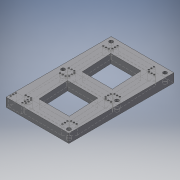
# Autodesk Inventor part: Segment
Saved by Autodesk Inventor 2016 SP2 (Build 200236200, 236)
## iProperties
Created: 2018-06-10
Part Number: Segment
Material: Generisch
Document SubType Name: Modeling
Designer: Nils
Density: 1 g/cm^3
Appearance: Vorgabe
Author: Nils
Autodesk Inventor part; units mm, degrees
ref_plane "YZ Plane" through (0, 0, 0) normal (1, 0, 0) x (0, 1, 0)
ref_plane "XZ Plane" through (0, 0, 0) normal (0, 1, 0) x (-1, 0, 0)
ref_plane "XY Plane" through (0, 0, 0) normal (0, 0, 1) x (1, 0, 0)
sketch "Skizze1" plane through (0, 0, 0) normal (0, 0, 1) x (1, 0, 0)
  line L0 (42.6168, 71.3457) -> (42.6168, -71.3457) projected
  line L1 (42.6168, -71.3457) -> (-42.6168, -71.3457) projected
  line L2 (-42.6168, -71.3457) -> (-42.6168, 71.3457) projected
  line L3 (-42.6168, 71.3457) -> (42.6168, 71.3457) projected
  line L4 (-27.6168, 66.3457) -> (22.3832, 66.3457) construction
  line L5 (22.3832, 56.3457) -> (-27.6168, 56.3457) construction
  line L6 (-28.3239, 55.6386) -> (-25.7071, 5.7071) construction
  line L7 (25.7071, 5.7071) -> (23.0903, 55.6386) construction
  line L8 (-25, 5) -> (25, 5) construction
  line L9 (25, -5) -> (-25, -5) construction
  line L10 (-25.7071, -5.7071) -> (-23.0903, -55.6386) construction
  line L11 (-22.3832, -56.3457) -> (27.6168, -56.3457) construction
  line L12 (27.6168, -66.3457) -> (-22.3832, -66.3457) construction
  line L13 (28.3239, -55.6386) -> (25.7071, -5.7071) construction
  line L14 (-22.5832, -56.1457) -> (27.8168, -56.1457)
  line L15 (27.8168, -56.1457) -> (27.8168, -66.5457)
  line L16 (27.8168, -66.5457) -> (-22.5832, -66.5457)
  line L17 (-22.5832, -66.5457) -> (-22.5832, -56.1457)
  line L18 (-25.2, 5.2) -> (25.2, 5.2)
  line L19 (25.2, 5.2) -> (25.2, -5.2)
  line L20 (25.2, -5.2) -> (-25.2, -5.2)
  line L21 (-25.2, -5.2) -> (-25.2, 5.2)
  line L22 (-27.8168, 66.5457) -> (22.5832, 66.5457)
  line L23 (22.5832, 66.5457) -> (22.5832, 56.1457)
  line L24 (22.5832, 56.1457) -> (-27.8168, 56.1457)
  line L25 (-27.8168, 56.1457) -> (-27.8168, 66.5457)
  line L26 (-25.4969, 5.5178) -> (-28.1346, 55.8488)
  line L27 (-28.1346, 55.8488) -> (-38.5204, 55.3045)
  line L28 (-38.5204, 55.3045) -> (-35.8827, 4.9736)
  line L29 (-35.8827, 4.9736) -> (-25.4969, 5.5178)
  line L30 (-25.5178, -5.4969) -> (-35.9036, -6.0412)
  line L31 (-35.9036, -6.0412) -> (-33.2659, -56.3721)
  line L32 (-33.2659, -56.3721) -> (-22.8801, -55.8278)
  line L33 (-22.8801, -55.8278) -> (-25.5178, -5.4969)
  line L34 (28.1346, -55.8488) -> (38.5204, -55.3045)
  line L35 (38.5204, -55.3045) -> (35.8827, -4.9736)
  line L36 (35.8827, -4.9736) -> (25.4969, -5.5178)
  line L37 (25.4969, -5.5178) -> (28.1346, -55.8488)
  line L38 (22.8801, 55.8278) -> (25.5178, 5.4969)
  line L39 (25.5178, 5.4969) -> (35.9178, 6.042)
  line L40 (35.9178, 6.042) -> (33.2801, 56.3729)
  line L41 (33.2801, 56.3729) -> (22.8801, 55.8278)
  circle A0 centre (-34.6168, -63.3457) radius 4 construction
  line L42 (-24.4168, -57.8457) -> (-41.4168, -57.8457)
  line L43 (-41.4168, -57.8457) -> (-41.4168, -68.8457)
  line L44 (-41.4168, -68.8457) -> (-24.4168, -68.8457)
  line L45 (-24.4168, -68.8457) -> (-24.4168, -57.8457)
  line L46 (20.7354, -10.2) -> (-20.2645, -10.2)
  line L47 (-20.2645, -10.2) -> (-18.1186, -51.1457)
  line L48 (-18.1186, -51.1457) -> (22.8813, -51.1457)
  line L49 (22.8813, -51.1457) -> (20.7354, -10.2)
  line L50 (-22.8813, 51.1457) -> (-20.7354, 10.2)
  line L51 (-22.8813, 51.1457) -> (18.1186, 51.1457)
  line L52 (20.2645, 10.2) -> (-20.7354, 10.2)
  line L53 (18.1186, 51.1457) -> (20.2645, 10.2)
  point P0 (0, 0)
  dimension "d0" = 0.2
  dimension "d1" = 0.2
  dimension "d2" = 0.2
  dimension "d3" = 0.2
  dimension "d4" = 0.2
  dimension "d5" = 0.2
  dimension "d6" = 0.2
  dimension "d7" = 0.2
  dimension "d8" = 0.2
  dimension "d9" = 0.2
  dimension "d10" = 0.2
  dimension "d11" = 0.2
  dimension "d12" = 0.2
  dimension "d13" = 0.2
  dimension "d14" = 0.2
  dimension "d17" = 10.4
  dimension "d18" = 10.4
  dimension "d19" = 10.4
  dimension "d21" = 50.4
  dimension "d22" = 50.4
  dimension "d23" = 50.4
  dimension "d24" = 0.2
  dimension "d25" = 0.2
  dimension "d26" = 0.2
  dimension "d28" = 90
  dimension "d29" = 50.4
  dimension "d30" = 0.2
  dimension "d31" = 0.2
  dimension "d32" = 10.4
  dimension "d35" = 17
  dimension "d36" = 11
  dimension "d37" = 5.5
  dimension "d38" = 1.2
  dimension "d49" = 5
  dimension "d50" = 5
  dimension "d51" = 5
  dimension "d52" = 5
  dimension "d54" = 5
  dimension "d56" = 5
  dimension "d57" = 5
  dimension "d58" = 5
  constraints: 80 end point, 21 parallel, 10 perpendicular, 7 horizontal
  measures "d0" distance between parallel lines of L14 L11
  measures "d1" distance between parallel lines of L12 L16
  measures "d2" distance from line of L17 L12.end
  measures "d3" distance from line of L12.start L15
  measures "d4" distance between parallel lines of L9 L20
  measures "d5" distance between parallel lines of L8 L18
  measures "d6" distance from line of L19 L8.end
  measures "d7" distance from line of L9.end L21
  measures "d8" distance between parallel lines of L5 L24
  measures "d9" distance between parallel lines of L22 L4
  measures "d10" distance from line of L23 L5.start
  measures "d11" distance from line of L25 L5.end
  measures "d12" distance between parallel lines of L13 L37
  measures "d13" distance between parallel lines of L33 L10
  measures "d14" distance between parallel lines of L26 L6
  measures "d17" distance between parallel lines of L35 L37
  measures "d18" distance between parallel lines of L31 L33
  measures "d19" distance between parallel lines of L28 L26
  measures "d21" distance of L34.end L35.end
  measures "d22" distance of L30.end L31.end
  measures "d23" distance of L27.end L28.end
  measures "d24" distance from line of L32 L10.end
  measures "d25" distance from line of L34 L13.start
  measures "d26" distance from line of L29 L6.end
  measures "d28" angle of L40 L39
  measures "d29" distance of L39.end L40.end
  measures "d30" distance from line of L39 L7.start
  measures "d31" distance between parallel lines of L7 L38
  measures "d32" horizontal distance of L38.end L39.end
  measures "d35" distance of L43.end L44.end
  measures "d36" distance between parallel lines of L44 L42
  measures "d37" distance from line of L44 A0.centre
  measures "d38" distance between parallel lines of L2 L43
  measures "d49" distance between parallel lines of L49 L37
  measures "d50" distance between parallel lines of L33 L47
  measures "d51" distance between parallel lines of L14 L48
  measures "d52" distance between parallel lines of L20 L46
  measures "d54" distance between parallel lines of L26 L50
  measures "d56" distance between parallel lines of L53 L38
  measures "d57" distance between parallel lines of L24 L51
  measures "d58" distance between parallel lines of L52 L18
extrude "Extrusion1" add sketch "Skizze1" along normal blind 11 contours L0 L1 L2 L3 | L45 L44 L43 L42
sketch "Skizze2" plane through (0, 0, 0) normal (0, 0, -1) x (-1, 0, 0)
  line L0 (22.3832, -56.3457) -> (27.3832, -61.3457) construction
  line L1 (27.3832, -61.3457) -> (22.3832, -66.3457) construction
  line L2 (22.3832, -66.3457) -> (-27.6168, -66.3457) construction
  line L3 (-27.6168, -66.3457) -> (-32.6168, -61.3457) construction
  line L4 (-32.6168, -61.3457) -> (-27.6168, -56.3457) construction
  line L5 (-27.6168, -56.3457) -> (22.3832, -56.3457) construction
  line L6 (-25, 5) -> (25, 5) construction
  line L7 (25, 5) -> (30, 0) construction
  line L8 (30, 0) -> (25, -5) construction
  line L9 (25, -5) -> (-25, -5) construction
  line L10 (-25, -5) -> (-30, 0) construction
  line L11 (-30, 0) -> (-25, 5) construction
  line L12 (-22.3832, 66.3457) -> (27.6168, 66.3457) construction
  line L13 (27.6168, 66.3457) -> (32.6168, 61.3457) construction
  line L14 (32.6168, 61.3457) -> (27.6168, 56.3457) construction
  line L15 (27.6168, 56.3457) -> (-22.3832, 56.3457) construction
  line L16 (-22.3832, 56.3457) -> (-27.3832, 61.3457) construction
  line L17 (-27.3832, 61.3457) -> (-22.3832, 66.3457) construction
  line L18 (23.0903, -55.6386) -> (25.7071, -5.7071) construction
  line L19 (25.7071, -5.7071) -> (30.7071, -0.7071) construction
  line L20 (30.7071, -0.7071) -> (35.7071, -5.7071) construction
  line L21 (35.7071, -5.7071) -> (33.0903, -55.6386) construction
  line L22 (33.0903, -55.6386) -> (28.0903, -60.6386) construction
  line L23 (28.0903, -60.6386) -> (23.0903, -55.6386) construction
  line L24 (-30.7071, -0.7071) -> (-25.7071, -5.7071) construction
  line L25 (-25.7071, -5.7071) -> (-28.3239, -55.6386) construction
  line L26 (-28.3239, -55.6386) -> (-33.3239, -60.6386) construction
  line L27 (-33.3239, -60.6386) -> (-38.3239, -55.6386) construction
  line L28 (-38.3239, -55.6386) -> (-35.7071, -5.7071) construction
  line L29 (-35.7071, -5.7071) -> (-30.7071, -0.7071) construction
  line L30 (35.7071, 5.7071) -> (30.7071, 0.7071) construction
  line L31 (30.7071, 0.7071) -> (25.7071, 5.7071) construction
  line L32 (25.7071, 5.7071) -> (28.3239, 55.6386) construction
  line L33 (28.3239, 55.6386) -> (33.3239, 60.6386) construction
  line L34 (33.3239, 60.6386) -> (38.3239, 55.6386) construction
  line L35 (38.3239, 55.6386) -> (35.7071, 5.7071) construction
  line L36 (-23.0903, 55.6386) -> (-25.7071, 5.7071) construction
  line L37 (-25.7071, 5.7071) -> (-30.7071, 0.7071) construction
  line L38 (-30.7071, 0.7071) -> (-35.7071, 5.7071) construction
  line L39 (-35.7071, 5.7071) -> (-33.0903, 55.6386) construction
  line L40 (-33.0903, 55.6386) -> (-28.0903, 60.6386) construction
  line L41 (-28.0903, 60.6386) -> (-23.0903, 55.6386) construction
  circle A0 centre (34.6168, -63.3457) radius 4 construction
  line L42 (-42.6168, -71.3457) -> (42.6168, -71.3457) construction
  line L43 (42.6168, -71.3457) -> (42.6168, 71.3457) construction
  line L44 (42.6168, 71.3457) -> (-42.6168, 71.3457) construction
  line L45 (-42.6168, 71.3457) -> (-42.6168, -71.3457) construction
  line L46 (-25.4969, -5.5178) -> (-30.7071, -0.3077)
  line L47 (-30.7071, -0.3077) -> (-35.3984, -4.9989)
  line L48 (-25.4969, -5.5178) -> (-35.8827, -4.9736) projected
  line L49 (-35.3984, -4.9989) -> (-35.8827, -4.9736)
  line L50 (-38.5204, -55.3045) -> (-28.1346, -55.8488) projected
  line L51 (-28.1346, -55.8488) -> (-33.3239, -61.038)
  line L52 (-33.3239, -61.038) -> (-38.5471, -55.8148)
  line L53 (-38.5471, -55.8148) -> (-38.5204, -55.3045)
  line L54 (-33.2801, 56.3729) -> (-22.8801, 55.8278) construction
  line L55 (-22.8801, 55.8278) -> (-25.5178, 5.4969) construction
  line L56 (-25.5178, 5.4969) -> (-35.9178, 6.042) construction
  line L57 (-35.9178, 6.042) -> (-33.2801, 56.3729) construction
  line L58 (-25.4969, -5.5178) -> (-28.1346, -55.8488) construction
  line L59 (-28.1346, -55.8488) -> (-38.5204, -55.3045) construction
  line L60 (-38.5204, -55.3045) -> (-35.8827, -4.9736) construction
  line L61 (-35.8827, -4.9736) -> (-25.4969, -5.5178) construction
  line L62 (22.8801, -55.8278) -> (25.5178, -5.4969) construction
  line L63 (25.5178, -5.4969) -> (35.9036, -6.0412) construction
  line L64 (35.9036, -6.0412) -> (33.2659, -56.3721) construction
  line L65 (33.2659, -56.3721) -> (22.8801, -55.8278) construction
  line L66 (35.8827, 4.9736) -> (25.4969, 5.5178) construction
  line L67 (25.4969, 5.5178) -> (28.1346, 55.8488) construction
  line L68 (28.1346, 55.8488) -> (38.5204, 55.3045) construction
  line L69 (38.5204, 55.3045) -> (35.8827, 4.9736) construction
  line L70 (-22.5832, 56.1457) -> (-22.5832, 66.5457) construction
  line L71 (-22.5832, 66.5457) -> (27.8168, 66.5457) construction
  line L72 (27.8168, 66.5457) -> (27.8168, 56.1457) construction
  line L73 (27.8168, 56.1457) -> (-22.5832, 56.1457) construction
  line L74 (-25.2, -5.2) -> (-25.2, 5.2) construction
  line L75 (-25.2, 5.2) -> (25.2, 5.2) construction
  line L76 (25.2, 5.2) -> (25.2, -5.2) construction
  line L77 (25.2, -5.2) -> (-25.2, -5.2) construction
  line L78 (-27.8168, -66.5457) -> (-27.8168, -56.1457) construction
  line L79 (-27.8168, -56.1457) -> (22.5832, -56.1457) construction
  line L80 (22.5832, -56.1457) -> (22.5832, -66.5457) construction
  line L81 (22.5832, -66.5457) -> (-27.8168, -66.5457) construction
  line L82 (-42.6168, 71.3457) -> (-42.6168, -71.3457) construction
  line L83 (-42.6168, -71.3457) -> (42.6168, -71.3457) construction
  line L84 (42.6168, -71.3457) -> (42.6168, 71.3457) construction
  line L85 (42.6168, 71.3457) -> (-42.6168, 71.3457) construction
  line L86 (22.5832, -56.1457) -> (-27.8168, -56.1457) projected
  line L87 (-27.8168, -56.1457) -> (-33.0168, -61.3457)
  line L88 (-33.0168, -61.3457) -> (-27.8168, -66.5457)
  line L89 (-27.8168, -66.5457) -> (22.5832, -66.5457) projected
  line L90 (-27.8168, -66.5457) -> (-27.8168, -56.1457)
  line L91 (22.5832, -66.5457) -> (22.5832, -56.1457) projected
  line L92 (22.5832, -66.5457) -> (27.7832, -61.3457)
  line L93 (27.7832, -61.3457) -> (22.5832, -56.1457)
  line L94 (22.5832, -56.1457) -> (22.5832, -66.5457)
  line L95 (22.8801, -55.8278) -> (33.2659, -56.3721) projected
  line L96 (22.8801, -55.8278) -> (28.0906, -61.0383)
  line L97 (28.0906, -61.0383) -> (32.7821, -56.3468)
  line L98 (33.2659, -56.3721) -> (35.9036, -6.0412) projected
  line L99 (33.2659, -56.3721) -> (32.7821, -56.3468)
  line L100 (35.9036, -6.0412) -> (25.5178, -5.4969) projected
  line L101 (25.5178, -5.4969) -> (30.7071, -0.3077)
  line L102 (30.7071, -0.3077) -> (35.9303, -5.5309)
  line L103 (35.9303, -5.5309) -> (35.9036, -6.0412)
  line L104 (35.9036, -6.0412) -> (25.5178, -5.4969)
  line L105 (25.2, -5.2) -> (30.4, 0)
  line L106 (30.4, 0) -> (25.2, 5.2)
  line L107 (-25.2, -5.2) -> (25.2, -5.2) projected
  line L108 (25.2, 5.2) -> (25.2, -5.2)
  line L109 (-25.2, -5.2) -> (-30.4, 0)
  line L110 (-30.4, 0) -> (-25.2, 5.2)
  line L111 (-25.5178, 5.4969) -> (-22.8801, 55.8278) projected
  line L112 (-25.5178, 5.4969) -> (-30.7074, 0.3074)
  line L113 (-30.7074, 0.3074) -> (-35.9439, 5.5439)
  line L114 (-35.9178, 6.042) -> (-25.5178, 5.4969) projected
  line L115 (-35.9439, 5.5439) -> (-35.9178, 6.042)
  line L116 (-35.9178, 6.042) -> (-25.5178, 5.4969)
  line L117 (-25.2, 5.2) -> (-25.2, -5.2) projected
  line L118 (-25.2, 5.2) -> (-25.2, -5.2)
  line L119 (25.4969, 5.5178) -> (30.7071, 0.3077)
  line L120 (30.7071, 0.3077) -> (35.3984, 4.9989)
  line L121 (25.4969, 5.5178) -> (35.8827, 4.9736) projected
  line L122 (38.5204, 55.3045) -> (35.8827, 4.9736) projected
  line L123 (35.8827, 4.9736) -> (35.3984, 4.9989)
  line L124 (28.1346, 55.8488) -> (25.4969, 5.5178) projected
  line L125 (35.3984, 4.9989) -> (25.4969, 5.5178)
  line L126 (-22.8801, 55.8278) -> (-28.0903, 61.038)
  line L127 (-28.0903, 61.038) -> (-32.7816, 56.3468)
  line L128 (-22.8801, 55.8278) -> (-33.2801, 56.3729) projected
  line L129 (-32.7816, 56.3468) -> (-22.8801, 55.8278)
  line L130 (-22.5832, 56.1457) -> (-27.7832, 61.3457)
  line L131 (-27.7832, 61.3457) -> (-22.5832, 66.5457)
  line L132 (-22.5832, 66.5457) -> (-22.5832, 56.1457) projected
  line L133 (-22.5832, 66.5457) -> (-22.5832, 56.1457)
  line L134 (-22.5832, 56.1457) -> (27.8168, 56.1457) projected
  line L135 (27.8168, 56.1457) -> (33.0168, 61.3457)
  line L136 (33.0168, 61.3457) -> (27.8168, 66.5457)
  line L137 (27.8168, 56.1457) -> (27.8168, 66.5457) projected
  line L138 (27.8168, 56.1457) -> (27.8168, 66.5457)
  line L139 (28.1346, 55.8488) -> (33.3239, 61.038)
  line L140 (33.3239, 61.038) -> (38.5471, 55.8148)
  line L141 (38.5471, 55.8148) -> (38.5204, 55.3045)
  line L142 (28.1346, 55.8488) -> (38.5204, 55.3045) projected
  line L143 (28.1346, 55.8488) -> (38.5204, 55.3045)
  point P0 (0, 0)
  dimension "d39" = 0.2825
  dimension "d40" = 0.2825
  dimension "d41" = 0.2825
  dimension "d42" = 0.2825
  dimension "d43" = 0.2825
  dimension "d44" = 0.2825
  dimension "d45" = 0.2825
  constraints: 92 end point, 21 perpendicular, 18 parallel, 9 collinear, 8 point on line, 1 vertical
  measures "d39" distance between parallel lines of L47 L29
  measures "d40" distance between parallel lines of L46 L24
  measures "d41" distance between parallel lines of L52 L27
  measures "d42" distance between parallel lines of L102 L20
  measures "d43" distance between parallel lines of L120 L30
  measures "d44" distance between parallel lines of L40 L127
  measures "d45" distance between parallel lines of L140 L34
extrude "Extrusion2" cut sketch "Skizze2" against normal blind 9 contours L48 L47 L46 | L50 L51 L52 L53 | L93 L92 L91 | L90 L88 L87 | L95 L97 L96 | L100 L101 L102 L103 | L108 L106 L105 | L109 L110 L117 | L112 L113 L115 L114 | L121 L120 L119 | L139 L140 L141 L142 | L128 L127 L126 | L130 L131 L132 | L137 L136 L135
sketch "Skizze3" plane through (0, 0, 0) normal (0, 0, -1) x (-1, 0, 0)
  circle A0 centre (34.6168, -63.3457) radius 4 projected
  line L0 (41.4168, -68.8457) -> (24.4168, -68.8457)
  line L1 (24.4168, -68.8457) -> (24.4168, -57.8457)
  line L2 (24.4168, -57.8457) -> (41.4168, -57.8457)
  line L3 (41.4168, -57.8457) -> (41.4168, -68.8457)
  line L4 (42.6168, -71.3457) -> (42.6168, 71.3457) projected
  line L5 (24.4168, -66.4092) -> (32.9803, -57.8457)
  line L6 (32.7821, -56.3468) -> (28.0906, -61.0383) projected
  point P0 (0, 0)
  dimension "d59" = 11
  dimension "d60" = 5.5
  dimension "d61" = 1.2
  dimension "d62" = 17
  dimension "d63" = 1.2
  constraints: 10 end point, 3 parallel, 2 point on line, 1 horizontal, 1 perpendicular
  measures "d59" distance of L2.end L0.start
  measures "d60" distance from line of L0 A0.centre
  measures "d61" distance between parallel lines of L4 L3
  measures "d62" distance of L0.start L0.end
  measures "d63" distance between parallel lines of L5 L6
extrude "Extrusion3" cut sketch "Skizze3" against normal blind 11 contours A0 | L0 L1 L5 L2 L3
sketch "Skizze4" plane through (0, 0, 11) normal (0, 0, 1) x (1, 0, 0)
  line L0 (-24.4168, -68.8457) -> (-41.4168, -68.8457) projected
  line L1 (-41.4168, -68.8457) -> (-24.4168, -68.8457)
  line L2 (-24.4168, -68.8457) -> (-24.4168, -57.8457)
  line L3 (-24.4168, -57.8457) -> (-41.4168, -57.8457)
  line L4 (-41.4168, -57.8457) -> (-41.4168, -68.8457)
  point P0 (0, 0)
  dimension "d66" = 11
  dimension "d67" = 17
  constraints: 8 end point, 2 parallel, 1 horizontal, 1 perpendicular
  measures "d66" distance of L1.end L2.end
  measures "d67" distance of L2.end L3.end
extrude "Extrusion4" cut sketch "Skizze4" against normal blind 4
sketch "Skizze5" plane through (0, 0, 9) normal (0, 0, -1) x (-1, 0, 0)
  line L0 (24.4168, -64.7121) -> (24.4168, -57.9793) projected
  line L1 (22.5832, -56.1457) -> (24.4168, -57.9793) projected
  line L2 (22.5832, -66.5457) -> (22.5832, -56.1457) projected
  line L3 (24.4168, -64.7121) -> (22.5832, -66.5457) projected
  line L4 (24.898, -57.8457) -> (31.2832, -57.8457) projected
  line L5 (32.7821, -56.3468) -> (31.2832, -57.8457) projected
  line L6 (22.8801, -55.8278) -> (32.7821, -56.3468) projected
  line L7 (24.898, -57.8457) -> (22.8801, -55.8278) projected
  point P0 (0, 0)
extrude "Extrusion5" add sketch "Skizze5" along normal blind 2
sketch "Skizze6" plane through (0, 0, 7) normal (0, 0, -1) x (-1, 0, 0)
  line L0 (24.4168, -64.7121) -> (24.4168, -57.9793) projected
  line L1 (22.5832, -56.1457) -> (24.4168, -57.9793) projected
  line L2 (22.5832, -56.1457) -> (22.5832, -66.5457) projected
  line L3 (24.4168, -64.7121) -> (22.5832, -66.5457) projected
  line L4 (24.898, -57.8457) -> (31.2832, -57.8457) projected
  line L5 (32.7821, -56.3468) -> (31.2832, -57.8457) projected
  line L6 (32.7821, -56.3468) -> (22.8801, -55.8278) projected
  line L7 (24.898, -57.8457) -> (22.8801, -55.8278) projected
  line L8 (27.7832, -61.3457) -> (22.5832, -66.5457) projected
  line L9 (22.5832, -56.1457) -> (27.7832, -61.3457) projected
  line L10 (32.7821, -56.3468) -> (28.0906, -61.0383) projected
  line L11 (28.0906, -61.0383) -> (22.8801, -55.8278) projected
  point P0 (0, 0)
extrude "Extrusion6" add sketch "Skizze6" along normal blind 1.5
chamfer "Fase1" distance 1.5 angle 45 2 edges at (-22.5832, -61.3457, 5.5) (-27.8311, -56.0873, 5.5)
sketch "Skizze7" plane through (0, 0, 11) normal (0, 0, 1) x (1, 0, 0)
  line L0 (42.6168, -71.3457) -> (42.6168, 71.3457) projected
  line L1 (-42.6168, -71.3457) -> (42.6168, -71.3457) projected
  line L2 (42.6168, 71.3457) -> (-42.6168, 71.3457)
  line L3 (-42.6168, 71.3457) -> (-42.6168, -71.3457)
  line L4 (-42.6168, -71.3457) -> (42.6168, -71.3457)
  line L5 (42.6168, -71.3457) -> (42.6168, 71.3457)
  line L6 (22.8813, -51.1457) -> (-18.1186, -51.1457) projected
  line L7 (-18.1186, -51.1457) -> (-20.2645, -10.2) projected
  line L8 (-20.2645, -10.2) -> (20.7354, -10.2) projected
  line L9 (20.7354, -10.2) -> (22.8813, -51.1457) projected
  line L10 (20.2645, 10.2) -> (-20.7354, 10.2) projected
  line L11 (-20.7354, 10.2) -> (-22.8813, 51.1457) projected
  line L12 (-22.8813, 51.1457) -> (18.1186, 51.1457) projected
  line L13 (18.1186, 51.1457) -> (20.2645, 10.2) projected
  point P0 (0, 0)
  constraints: 8 end point, 2 parallel, 1 horizontal, 1 perpendicular
extrude "Extrusion7" add sketch "Skizze7" along normal blind 1
sketch "Skizze8" plane through (0, 0, 11) normal (0, 0, -1) x (-1, 0, 0)
  line L0 (22.5832, -66.5457) -> (-27.8168, -66.5457) construction
  line L1 (22.0832, -66.5457) -> (22.0832, -56.1457) construction
  line L2 (-27.8168, -56.1457) -> (22.5832, -56.1457) construction
  line L3 (-27.3168, -66.5457) -> (-27.3168, -56.1457) construction
  line L4 (-25.4969, -5.5178) -> (-28.1346, -55.8488) construction
  line L5 (-28.1085, -55.3495) -> (-38.4942, -54.8052) construction
  line L6 (-35.8827, -4.9736) -> (-38.5204, -55.3045) construction
  line L7 (22.8801, -55.8278) -> (25.5178, -5.4969) construction
  line L8 (22.9063, -55.3285) -> (33.292, -55.8728) construction
  line L9 (35.9303, -5.5309) -> (33.2659, -56.3721) construction
  line L10 (41.4168, -68.8457) -> (24.4168, -68.8457) construction
  line L11 (24.9168, -68.8457) -> (24.9168, -57.8457) construction
  line L12 (32.9803, -57.8457) -> (24.4168, -57.8457) construction
  line L13 (40.9168, -68.8457) -> (40.9168, -57.8457) construction
  line L14 (32.9803, -57.8457) -> (41.4168, -57.8457) construction
  line L15 (-35.9088, -5.4729) -> (-25.5231, -6.0172) construction
  line L16 (25.2, -5.2) -> (-25.2, -5.2) construction
  line L17 (-24.7, -5.2) -> (-24.7, 5.2) construction
  line L18 (-25.2, 5.2) -> (25.2, 5.2) construction
  line L19 (24.7, -5.2) -> (24.7, 5.2) construction
  line L20 (25.4917, -5.9962) -> (35.8774, -6.5405) construction
  line L21 (-33.2801, 56.3729) -> (-35.9178, 6.042) construction
  line L22 (-35.8917, 6.5413) -> (-25.4917, 5.9962) construction
  line L23 (-25.5178, 5.4969) -> (-22.8801, 55.8278) construction
  line L24 (25.4969, 5.5178) -> (28.1346, 55.8488) construction
  line L25 (25.5231, 6.0172) -> (35.9088, 5.4729) construction
  line L26 (38.5471, 55.8148) -> (35.8827, 4.9736) construction
  line L27 (-22.9063, 55.3285) -> (-33.3063, 55.8736) construction
  line L28 (28.1085, 55.3495) -> (38.4942, 54.8052) construction
  line L29 (27.8168, 56.1457) -> (-22.5832, 56.1457) construction
  line L30 (27.3168, 56.1457) -> (27.3168, 66.5457) construction
  line L31 (-22.5832, 66.5457) -> (27.8168, 66.5457) construction
  line L32 (-22.0832, 56.1457) -> (-22.0832, 66.5457) construction
  line L33 (-22.5832, 66.5457) -> (-22.5832, 56.1457) construction
  line L34 (-22.8801, 55.8278) -> (-32.7816, 56.3468) construction
  line L35 (27.8168, 56.1457) -> (27.8168, 66.5457) construction
  line L36 (38.5204, 55.3045) -> (28.1346, 55.8488) construction
  line L37 (25.4969, 5.5178) -> (35.3984, 4.9989) construction
  line L38 (-35.9178, 6.042) -> (-25.5178, 5.4969) construction
  line L39 (-25.2, 5.2) -> (-25.2, -5.2) construction
  line L40 (-25.4969, -5.5178) -> (-35.3984, -4.9989) construction
  line L41 (35.9036, -6.0412) -> (25.5178, -5.4969) construction
  line L42 (-38.5204, -55.3045) -> (-28.1346, -55.8488) construction
  line L43 (-27.8168, -56.1457) -> (-27.8168, -66.5457) construction
  line L44 (22.5832, -66.5457) -> (22.5832, -56.1457) construction
  line L45 (22.8801, -55.8278) -> (33.2659, -56.3721) construction
  line L46 (24.4168, -68.8457) -> (24.4168, -66.4092) construction
  line L47 (41.4168, -57.8457) -> (41.4168, -68.8457) construction
  line L48 (25.2, -5.2) -> (25.2, 5.2) construction
  circle A0 centre (-33.3014, -55.0773) radius 1
  circle A1 centre (-36.8014, -54.8939) radius 1
  circle A2 centre (-29.8014, -55.2607) radius 1
  circle A3 centre (-27.3168, -61.3457) radius 1
  circle A4 centre (-27.3168, -57.8457) radius 1
  circle A5 centre (-27.3168, -64.8457) radius 1
  circle A6 centre (22.0832, -61.3457) radius 1
  circle A7 centre (22.0832, -57.8457) radius 1
  circle A8 centre (22.0832, -64.8457) radius 1
  circle A9 centre (40.9168, -63.3457) radius 1
  circle A10 centre (40.9168, -66.8457) radius 1
  circle A11 centre (40.9168, -59.8457) radius 1
  circle A12 centre (24.9168, -66.8457) radius 1
  circle A13 centre (24.9168, -59.8457) radius 1
  circle A14 centre (24.9168, -63.3457) radius 1
  circle A15 centre (28.0992, -55.6007) radius 1
  circle A16 centre (31.5992, -55.7841) radius 1
  circle A17 centre (24.5992, -55.4172) radius 1
  circle A18 centre (30.6846, -6.2684) radius 1
  circle A19 centre (27.1846, -6.0849) radius 1
  circle A20 centre (34.1846, -6.4518) radius 1
  circle A21 centre (24.7, 0) radius 1
  circle A22 centre (24.7, 3.5) radius 1
  circle A23 centre (24.7, -3.5) radius 1
  circle A24 centre (30.716, 5.745) radius 1
  circle A25 centre (34.216, 5.5616) radius 1
  circle A26 centre (27.216, 5.9284) radius 1
  circle A27 centre (-30.716, -5.745) radius 1
  circle A28 centre (-27.216, -5.9284) radius 1
  circle A29 centre (-34.216, -5.5616) radius 1
  circle A30 centre (-24.7, 0) radius 1
  circle A31 centre (-24.7, -3.5) radius 1
  circle A32 centre (-24.7, 3.5) radius 1
  circle A33 centre (-30.6917, 6.2687) radius 1
  circle A34 centre (-27.1917, 6.0853) radius 1
  circle A35 centre (-34.1917, 6.4522) radius 1
  circle A36 centre (-28.1063, 55.601) radius 1
  circle A37 centre (-24.6063, 55.4176) radius 1
  circle A38 centre (-31.6063, 55.7845) radius 1
  circle A39 centre (-22.0832, 61.3457) radius 1
  circle A40 centre (-22.0832, 57.8457) radius 1
  circle A41 centre (-22.0832, 64.8457) radius 1
  circle A42 centre (27.3168, 61.3457) radius 1
  circle A43 centre (27.3168, 64.8457) radius 1
  circle A44 centre (27.3168, 57.8457) radius 1
  circle A45 centre (33.3014, 55.0773) radius 1
  circle A46 centre (36.8014, 54.8939) radius 1
  circle A47 centre (29.8014, 55.2607) radius 1
  point P0 (0, 0)
  dimension "d79" = 0.5
  dimension "d80" = 0.5
  dimension "d81" = 0.5
  dimension "d82" = 0.5
  dimension "d83" = 0.5
  dimension "d84" = 0.5
  dimension "d85" = 0.5
  dimension "d86" = 0.5
  dimension "d87" = 0.5
  dimension "d88" = 0.5
  dimension "d89" = 0.5
  dimension "d90" = 0.5
  dimension "d91" = 0.5
  dimension "d92" = 0.5
  dimension "d93" = 0.5
  dimension "d94" = 0.5
  dimension "d95" = 2
  dimension "d96" = 2
  dimension "d97" = 2
  dimension "d98" = 2
  dimension "d99" = 2
  dimension "d100" = 2
  dimension "d101" = 2
  dimension "d102" = 2
  dimension "d103" = 2
  dimension "d104" = 2
  dimension "d105" = 2
  dimension "d106" = 2
  dimension "d107" = 2
  dimension "d108" = 2
  dimension "d109" = 2
  dimension "d110" = 2
  dimension "d111" = 2
  dimension "d112" = 2
  dimension "d113" = 2
  dimension "d114" = 2
  dimension "d115" = 2
  dimension "d116" = 2
  dimension "d117" = 2
  dimension "d118" = 2
  dimension "d119" = 2
  dimension "d120" = 2
  dimension "d121" = 2
  dimension "d122" = 2
  dimension "d123" = 2
  dimension "d124" = 2
  dimension "d125" = 2
  dimension "d126" = 2
  dimension "d127" = 2
  dimension "d128" = 2
  dimension "d129" = 2
  dimension "d130" = 2
  dimension "d131" = 2
  dimension "d132" = 2
  dimension "d133" = 2
  dimension "d134" = 2
  dimension "d135" = 2
  dimension "d136" = 2
  dimension "d137" = 2
  dimension "d138" = 2
  dimension "d139" = 2
  dimension "d140" = 2
  dimension "d141" = 2
  dimension "d142" = 2
  constraints: 64 point on line, 48 centre point, 32 end point, 16 midpoint, 14 parallel, 1 vertical
  measures "d79" distance between parallel lines of L33 L32
  measures "d80" distance between parallel lines of L34 L27
  measures "d81" distance between parallel lines of L35 L30
  measures "d82" distance between parallel lines of L36 L28
  measures "d83" distance between parallel lines of L37 L25
  measures "d84" distance between parallel lines of L38 L22
  measures "d85" distance between parallel lines of L39 L17
  measures "d86" distance between parallel lines of L40 L15
  measures "d87" distance between parallel lines of L41 L20
  measures "d88" distance between parallel lines of L42 L5
  measures "d89" distance between parallel lines of L43 L3
  measures "d90" distance between parallel lines of L44 L1
  measures "d91" distance between parallel lines of L45 L8
  measures "d92" distance between parallel lines of L46 L11
  measures "d93" distance between parallel lines of L47 L13
  measures "d94" distance between parallel lines of L48 L19
  measures "d95" diameter of A0
  measures "d96" diameter of A1
  measures "d97" diameter of A2
  measures "d98" diameter of A4
  measures "d99" diameter of A3
  measures "d100" diameter of A5
  measures "d101" diameter of A8
  measures "d102" diameter of A6
  measures "d103" diameter of A7
  measures "d104" diameter of A15
  measures "d105" diameter of A17
  measures "d106" diameter of A16
  measures "d107" diameter of A13
  measures "d108" diameter of A14
  measures "d109" diameter of A12
  measures "d110" diameter of A10
  measures "d111" diameter of A9
  measures "d112" diameter of A11
  measures "d113" diameter of A18
  measures "d114" diameter of A20
  measures "d115" diameter of A19
  measures "d116" diameter of A23
  measures "d117" diameter of A21
  measures "d118" diameter of A22
  measures "d119" diameter of A26
  measures "d120" diameter of A24
  measures "d121" diameter of A25
  measures "d122" diameter of A28
  measures "d123" diameter of A27
  measures "d124" diameter of A29
  measures "d125" diameter of A31
  measures "d126" diameter of A30
  measures "d127" diameter of A32
  measures "d128" diameter of A34
  measures "d129" diameter of A33
  measures "d130" diameter of A35
  measures "d131" diameter of A38
  measures "d132" diameter of A36
  measures "d133" diameter of A37
  measures "d134" diameter of A40
  measures "d135" diameter of A39
  measures "d136" diameter of A41
  measures "d137" diameter of A44
  measures "d138" diameter of A42
  measures "d139" diameter of A43
  measures "d140" diameter of A47
  measures "d141" diameter of A45
  measures "d142" diameter of A46
extrude "Extrusion8" cut sketch "Skizze8" against normal blind 1
sketch "Skizze9" plane through (0, 0, 0) normal (0, 0, -1) x (-1, 0, 0)
  line L0 (42.6168, -71.3457) -> (42.6168, 71.3457) construction
  line L1 (-42.6168, -71.3457) -> (42.6168, -71.3457) construction
  line L2 (-42.6168, 71.3457) -> (-42.6168, -71.3457) construction
  line L3 (42.6168, 71.3457) -> (-42.6168, 71.3457) construction
  circle A0 centre (-36.6168, 65.3457) radius 2.5
  circle A1 centre (36.6168, 65.3457) radius 2.5
  circle A2 centre (-36.6168, 0) radius 2.5
  circle A3 centre (36.6168, 0) radius 2.5
  circle A4 centre (-37.6168, -66.3457) radius 2.5
  point P0 (0, 0)
  dimension "d177" = 5
  dimension "d178" = 5
  dimension "d179" = 5
  dimension "d180" = 5
  dimension "d181" = 5
  dimension "d182" = 6
  dimension "d183" = 6
  dimension "d184" = 6
  dimension "d185" = 6
  dimension "d186" = 6
  dimension "d187" = 6
  dimension "d188" = 71.3457
  dimension "d189" = 71.3457
  dimension "d190" = 5
  dimension "d191" = 5
  constraints: 5 centre point
  measures "d177" diameter of A0
  measures "d178" diameter of A1
  measures "d179" diameter of A2
  measures "d180" diameter of A3
  measures "d181" diameter of A4
  measures "d182" distance from line of L3 A0.centre
  measures "d183" distance from line of L2 A0.centre
  measures "d184" distance from line of L3 A1.centre
  measures "d185" distance from line of L0 A1.centre
  measures "d186" distance from line of L2 A2.centre
  measures "d187" distance from line of L0 A3.centre
  measures "d188" distance from line of L3 A2.centre
  measures "d189" distance from line of L3 A3.centre
  measures "d190" distance from line of L1 A4.centre
  measures "d191" distance from line of L2 A4.centre
extrude "Extrusion9" cut sketch "Skizze9" against normal blind 3
sketch "Skizze10" plane through (0, 0, 12) normal (0, 0, 1) x (1, 0, 0)
  circle A0 centre (-36.6168, 0) radius 2.5 projected
  circle A1 centre (37.6168, -66.3457) radius 2.5 projected
  circle A2 centre (36.6168, 0) radius 2.5 projected
  circle A3 centre (36.6168, 65.3457) radius 2.5 projected
  circle A4 centre (-36.6168, 65.3457) radius 2.5 projected
  point P0 (0, 0)
extrude "Extrusion10" cut sketch "Skizze10" against normal blind 3
sketch "Skizze12" plane through (0, 0, 0) normal (0, 0, -1) x (-1, 0, 0)
  line L0 (-35.3984, -4.9989) -> (-30.7071, -0.3077) projected
  line L1 (-30.8485, -0.4491) -> (-25.1859, -6.1117)
  line L2 (-25.1859, -6.1117) -> (-24.5957, -5.5214)
  line L3 (-24.5957, -5.5214) -> (-30.1172, 0)
  line L4 (-30.1172, 0) -> (-24.2907, 5.8264)
  line L5 (-24.2907, 5.8264) -> (-24.8809, 6.4167)
  line L6 (-24.8809, 6.4167) -> (-31.2976, 0)
  line L7 (-31.2976, 0) -> (-30.6583, -0.6393)
  line L8 (-25.5178, 5.4969) -> (-30.7074, 0.3074) projected
  line L9 (-30.4, 0) -> (-25.2, 5.2) projected
  line L10 (-25.2, -5.2) -> (-30.4, 0) projected
  line L11 (-30.7071, -0.3077) -> (-25.4969, -5.5178) projected
  line L12 (24.6488, -6.6488) -> (31.2976, 0)
  line L13 (31.2976, 0) -> (24.6488, 6.6488)
  line L14 (24.6488, 6.6488) -> (24.0586, 6.0586)
  line L15 (24.0586, 6.0586) -> (30.1172, 0)
  line L16 (30.1172, 0) -> (24.0586, -6.0586)
  line L17 (24.0586, -6.0586) -> (24.6488, -6.6488)
  line L18 (30.7071, 0.3077) -> (25.4969, 5.5178) projected
  line L19 (25.2, 5.2) -> (30.4, 0) projected
  line L20 (30.4, 0) -> (25.2, -5.2) projected
  line L21 (25.5178, -5.4969) -> (30.7071, -0.3077) projected
  line L22 (-28.8773, 61.5422) -> (-21.4578, 54.1227)
  line L23 (-21.4578, 54.1227) -> (-20.8676, 54.7129)
  line L24 (-20.8676, 54.7129) -> (-28.2871, 62.1324)
  line L25 (-28.2871, 62.1324) -> (-28.8773, 61.5422)
  line L26 (-28.0903, 61.038) -> (-22.8801, 55.8278) projected
  line L27 (-22.5832, 56.1457) -> (-27.7832, 61.3457) projected
  line L28 (26.326, 54.9378) -> (33.3326, 61.9443)
  line L29 (33.3326, 61.9443) -> (33.9228, 61.3541)
  line L30 (33.9228, 61.3541) -> (26.9162, 54.3475)
  line L31 (26.9162, 54.3475) -> (26.326, 54.9378)
  line L32 (33.0168, 61.3457) -> (27.8168, 56.1457) projected
  line L33 (28.1346, 55.8488) -> (33.3239, 61.038) projected
  line L34 (-34.2313, -61.6626) -> (-26.7988, -54.2301)
  line L35 (-26.7988, -54.2301) -> (-26.2086, -54.8203)
  line L36 (-26.2086, -54.8203) -> (-33.6411, -62.2528)
  line L37 (-33.6411, -62.2528) -> (-34.2313, -61.6626)
  line L38 (-28.1346, -55.8488) -> (-33.3239, -61.038) projected
  line L39 (-33.0168, -61.3457) -> (-27.8168, -56.1457) projected
  point P0 (0, 0)
  dimension "d197" = 0.2
  dimension "d198" = 0.2
  dimension "d199" = 0.2
  dimension "d200" = 0.2
  dimension "d201" = 0.2
  dimension "d202" = 0.2
  dimension "d203" = 0.2
  dimension "d204" = 0.2
  dimension "d205" = 0.2
  dimension "d206" = 0.2
  dimension "d207" = 0.2
  dimension "d208" = 0.2
  dimension "d209" = 0.2
  dimension "d210" = 0.2
  constraints: 50 end point, 17 perpendicular, 4 parallel, 2 point on line
  measures "d197" distance between parallel lines of L8 L6
  measures "d198" distance between parallel lines of L9 L4
  measures "d199" distance between parallel lines of L10 L3
  measures "d200" distance between parallel lines of L11 L1
  measures "d201" distance between parallel lines of L13 L18
  measures "d202" distance between parallel lines of L19 L15
  measures "d203" distance between parallel lines of L20 L16
  measures "d204" distance between parallel lines of L21 L12
  measures "d205" distance between parallel lines of L26 L22
  measures "d206" distance between parallel lines of L27 L24
  measures "d207" distance between parallel lines of L32 L28
  measures "d208" distance between parallel lines of L30 L33
  measures "d209" distance between parallel lines of L38 L34
  measures "d210" distance between parallel lines of L39 L36
extrude "Extrusion11" add sketch "Skizze12" against normal blind 9
sketch "Skizze13" plane through (0, 0, 0) normal (0, 0, -1) x (-1, 0, 0)
  line L0 (20.5773, -54.4227) -> (21.1676, -53.8324)
  line L1 (21.1676, -53.8324) -> (28.1676, -60.8324)
  line L2 (28.1676, -60.8324) -> (28.232, -60.8969)
  line L3 (32.7821, -56.3468) -> (28.0906, -61.0383) projected
  line L4 (28.232, -60.8969) -> (27.6418, -61.4871)
  line L5 (27.7832, -61.3457) -> (22.5832, -66.5457) projected
  line L6 (27.6418, -61.4871) -> (20.5773, -54.4227)
  line L7 (22.5832, -56.1457) -> (27.7832, -61.3457) projected
  line L8 (22.8801, -55.8278) -> (24.4652, -57.413) projected
  point P0 (0, 0)
  dimension "d213" = 0.2
  dimension "d214" = 0.2
  constraints: 10 end point, 3 point on line, 1 parallel, 1 perpendicular
  measures "d213" distance between parallel lines of L8 L1
  measures "d214" distance between parallel lines of L7 L6
extrude "Extrusion12" add sketch "Skizze13" against normal blind 7
equation "\"d0\" = d2"
equation "\"d1\" = d2"
equation "\"d3\" = d2"
equation "\"d4\" = d2"
equation "\"d5\" = d2"
equation "\"d6\" = d2"
equation "\"d7\" = d2"
equation "\"d8\" = d2"
equation "\"d9\" = d2"
equation "\"d10\" = d2"
equation "\"d11\" = d2"
equation "\"d12\" = d2"
equation "\"d13\" = d2"
equation "\"d14\" = d2"
equation "\"d17\" = d16"
equation "\"d18\" = d16"
equation "\"d19\" = d16"
equation "\"d21\" = d20"
equation "\"d22\" = d20"
equation "\"d23\" = d20"
equation "\"d24\" = d2"
equation "\"d25\" = d2"
equation "\"d26\" = d2"
equation "\"d30\" = d2"
equation "\"d31\" = d2"
equation "\"d50\" = d49"
equation "\"d51\" = d49"
equation "\"d52\" = d49"
equation "\"d54\" = d49"
equation "\"d39\" = d40"
equation "\"d41\" = d40"
equation "\"d42\" = d40"
equation "\"d43\" = d40"
equation "\"d44\" = d40"
equation "\"d45\" = d40"
equation "\"d16\" = 10.4"
equation "\"d20\" = 50.4"
